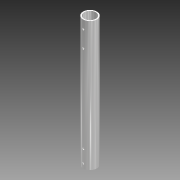
# Autodesk Inventor part: FE-120-002 Top Connector Bar
Saved by Autodesk Inventor 2021 (Build 250183000, 183)
## iProperties
Created: 2021-01-11
Part Number: FE-120-002 Top Connector Bar
Material: Aluminum 6061
Document SubType Name: Modeling
Density: 2.7 g/cm^3
Appearance: Aluminum - Dark
Autodesk Inventor part; units mm, degrees
ref_plane "YZ Plane" through (0, 0, 0) normal (1, 0, 0) x (0, 1, 0)
ref_plane "XZ Plane" through (0, 0, 0) normal (0, 1, 0) x (-1, 0, 0)
ref_plane "XY Plane" through (0, 0, 0) normal (0, 0, 1) x (1, 0, 0)
sketch "Sketch1" plane through (0, 0, 0) normal (0, 1, 0) x (-1, 0, 0)
  circle A0 centre (0, 0) radius 21.082
  circle A1 centre (0, 0) radius 17.526
  dimension "d0" = 42.164
  dimension "d1" = 35.052
  constraints: 2 centre point, 2 coincident
  measures "d0" diameter of A0
  measures "d1" diameter of A1
extrude "Extrusion1" add sketch "Sketch1" along normal mid plane 393.7
sketch "Sketch3" plane through (0, 0, 0) normal (0, 0, 1) x (1, 0, 0)
  circle A0 centre (0, 171.45) radius 3.175
  circle A1 centre (0, 120.65) radius 3.175
  line L0 (21.082, 196.85) -> (-21.082, 196.85) projected
  circle A2 centre (0, -182.5625) radius 3.175
  circle A3 centre (0, -144.4625) radius 3.175
  line L1 (-21.082, -196.85) -> (21.082, -196.85) projected
  point P0 (0, 0)
  dimension "d10" = 25.4
  dimension "d11" = 76.2
  dimension "d12" = 6.35
  dimension "d15" = 38.1
  dimension "d16" = 14.2875
  constraints: 4 centre point, 4 vertical alignment, 3 equal radius
  measures "d10" distance from line of A0.centre L0
  measures "d11" distance from line of A1.centre L0
  measures "d12" diameter of A0
  measures "d15" distance of A2.centre A3.centre
  measures "d16" distance from line of A2.centre L1
extrude "Extrusion3" cut sketch "Sketch3" against normal through all both and the other way through all
body "Solid1"
